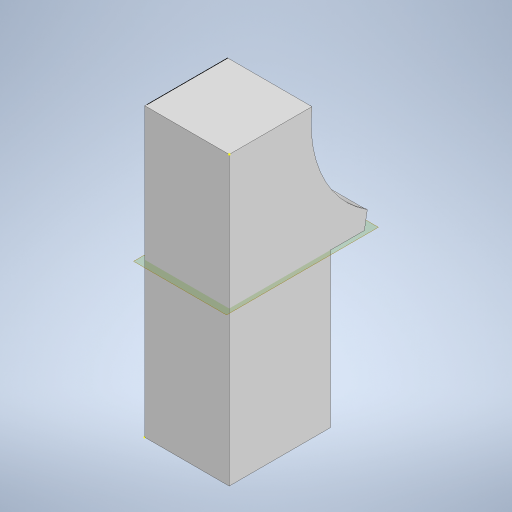
# Autodesk Inventor part: Pièce1
Saved by Autodesk Inventor 2023.1 (Build 271208000, 208)
## iProperties
Created: 2022-09-20
Part Number: Pièce1
Material: Générique
Document SubType Name: Sheet Metal
Designer: guiki
Density: 1 g/cm^3
Sheet Metal Rule: Par défaut_mm
Appearance: Par défaut
Author: guiki
Autodesk Inventor part; units mm, degrees
ref_plane "YZ Plane" through (0, 0, 0) normal (1, 0, 0) x (0, 1, 0)
ref_plane "XZ Plane" through (0, 0, 0) normal (0, 1, 0) x (-1, 0, 0)
ref_plane "XY Plane" through (0, 0, 0) normal (0, 0, 1) x (1, 0, 0)
sketch "Esquisse1" plane through (0, 0, 0) normal (0, 1, 0) x (-1, 0, 0)
  line L0 (0, 0) -> (500, 0)
  line L1 (500, 0) -> (500, -600)
  line L2 (500, -600) -> (0, -600)
  line L3 (0, -600) -> (0, 0)
  dimension "d0" = 500
  dimension "d1" = 600
  constraints: 8 end point, 2 parallel, 1 horizontal, 1 perpendicular
  measures "d0" distance of L1.end L2.end
  measures "d1" distance of L0.end L1.end
extrude "Extrusion1" add sketch "Esquisse1" along normal blind 1700
sketch "Esquisse3" plane through (0, 1700, 0) normal (0, 1, 0) x (1, 0, 0)
  line L0 (-500, 600) -> (-500, 0) projected
  line L1 (0, 600) -> (-500, 600) projected
  line L2 (-500, 13.2496) -> (0, 13.2496)
  line L3 (0, 13.2496) -> (0, 600)
  line L4 (0, 600) -> (-500, 600)
  line L5 (-500, 600) -> (-500, 13.2496)
  point P0 (0, 0)
  constraints: 8 end point, 2 parallel, 1 horizontal, 1 perpendicular, 1 point on line
extrude "Extrusion2" cut sketch "Esquisse3" against normal blind 790
sketch "Esquisse4" plane through (0, 910, 0) normal (0, 1, 0) x (1, 0, 0)
  line L0 (0, 13.2496) -> (-500, 13.2496) projected
  line L1 (0, 13.2496) -> (-10, 13.2496)
  line L2 (0, 600) -> (-500, 600) projected
  line L3 (-500, 600) -> (-490, 600)
  line L4 (-490, 600) -> (-490, 590)
  line L5 (-490, 590) -> (-10, 590)
  line L6 (-10, 590) -> (-10, 13.2496)
  line L7 (-10, 13.2496) -> (-490, 13.2496)
  line L8 (-490, 13.2496) -> (-490, 590)
  point P0 (0, 0)
  dimension "d7" = 10
  dimension "d8" = 10
  dimension "d9" = 10
  constraints: 14 end point, 2 parallel, 2 perpendicular, 2 point on line, 1 horizontal
  measures "d7" distance of L0.start L1.end
  measures "d8" distance of L2.end L3.end
  measures "d9" distance of L3.end L4.end
extrude "Extrusion3" cut sketch "Esquisse4" against normal blind 800
sketch "Esquisse5" plane through (0, 0, 0) normal (1, 0, 0) x (0, 0, -1)
  line L0 (600, 0) -> (600, 910) projected
  line L1 (600, 910) -> (800, 910)
  line L2 (800, 910) -> (817.3648, 1008.4808)
  line L3 (0, 0) -> (0, 1700) projected
  line L4 (0, 1700) -> (490, 1700)
  arc A0 (490, 1700) -> (817.3648, 1008.4808) centre (1204.9924, 1615.2302) ccw
  line L5 (13.2496, 1700) -> (13.2496, 910) projected
  line L6 (13.2496, 1700) -> (13.2496, 910)
  line L7 (13.2496, 910) -> (590, 910) projected
  line L8 (800, 910) -> (13.2496, 910)
  dimension "d12" = 200
  dimension "d13" = 100
  dimension "d14" = 100
  dimension "d15" = 490
  dimension "d16" = 720
  constraints: 10 end point, 3 horizontal, 2 point on circle, 1 centre point, 1 vertical
  measures "d12" distance of L0.end L1.end
  measures "d13" distance of L1.end L2.end
  measures "d14" angle of L2 L1
  measures "d15" distance of L3.end L4.end
  measures "d16" radius of A0
extrude "Extrusion4" add sketch "Esquisse5" against normal blind 10
sketch "Esquisse6" plane through (-500, 0, -600) normal (-1, 0, 0) x (0, 0, 1)
  line L0 (0, 0) -> (0, 910) projected
  line L1 (0, 910) -> (-200, 910) projected
  line L2 (0, 910) -> (-200, 910)
  line L3 (-200, 910) -> (-217.3648, 1008.4808)
  line L4 (586.7504, 910) -> (586.7504, 110) projected
  line L5 (0, 910) -> (586.7504, 910)
  line L6 (586.7504, 1700) -> (110, 1700) projected
  line L7 (586.7504, 910) -> (586.7504, 1700)
  line L8 (586.7504, 1700) -> (110, 1700)
  arc A0 (-217.3648, 1008.4808) -> (110, 1700) centre (-604.9924, 1615.2302) ccw
  point P0 (600, 0)
  dimension "d19" = 100
  dimension "d20" = 100
  constraints: 10 end point, 2 horizontal, 2 point on circle, 1 centre point, 1 collinear, 1 perpendicular
  measures "d19" distance of L1.end L3.end
  measures "d20" angle of L2 L3
sketch "Esquisse7" plane through (-500, 0, -600) normal (-1, 0, 0) x (0, 0, 1)
  line L0 (586.7504, 1700) -> (110, 1700) projected
  line L1 (110, 1700) -> (586.7504, 1700)
  line L2 (0, 0) -> (0, 910) projected
  line L3 (586.7504, 910) -> (10, 910) projected
  line L4 (0, 910) -> (586.7504, 910)
  line L5 (586.7504, 910) -> (586.7504, 1700)
  line L6 (0, 910) -> (-200, 910) projected
  line L7 (0, 910) -> (-200, 910)
  line L8 (-217.3648, 1008.4808) -> (-200, 910) projected
  line L9 (-200, 910) -> (-217.3648, 1008.4808)
  point P0 (600, 0)
  constraints: 10 end point, 2 collinear, 2 horizontal, 1 perpendicular
extrude "Extrusion5" add sketch "Esquisse6" against normal blind 10
ref_plane "Plan de construction1" through (0, 910, -800) normal (0, -1, 0) x (1, 0, 0)
sketch "Esquisse8" plane through (0, 910, -800) normal (0, -1, 0) x (1, 0, 0)
  line L0 (-10, 0) -> (-10, 200) projected
  line L1 (0, 200) -> (-500, 200) projected
  line L2 (-10, 0) -> (-490, 0)
  line L3 (-490, 0) -> (-490, 200)
  line L4 (-490, 200) -> (-10, 200)
  line L5 (-10, 200) -> (-10, 0)
  point P0 (0, 800)
  dimension "d23" = 480
  constraints: 8 end point, 2 parallel, 1 horizontal, 1 perpendicular, 1 point on line
  measures "d23" distance of L3.end L4.end
extrude "Extrusion6" add sketch "Esquisse8" against normal blind 10
sketch "Esquisse9" plane through (-490, 1008.4808, -817.3648) normal (0, -0.1736, -0.9848) x (-1, 0, 0)
  line L0 (-480, 541.3803) -> (-480, -1024.464) projected
  line L1 (0, -90.1519) -> (0, -100) projected
  line L2 (-480, -2.3513) -> (0, -2.3513)
  line L3 (0, -2.3513) -> (0, -90.1519)
  line L4 (0, -90.1519) -> (-480, -90.1519)
  line L5 (-480, -90.1519) -> (-480, -2.3513)
  point P0 (-490, -1135.0936)
  constraints: 8 end point, 2 parallel, 1 horizontal, 1 perpendicular, 1 point on line
extrude "Extrusion7" add sketch "Esquisse9" against normal blind 10
sketch "Esquisse10" plane through (0, 1700, 0) normal (0, 1, 0) x (1, 0, 0)
  point P0 (0, 0)
sketch "Esquisse11" plane through (0, 1700, 0) normal (0, 1, 0) x (1, 0, 0)
  line L0 (-500, 490) -> (-490, 490) projected
  line L1 (-490, 490) -> (-490, 10)
  line L2 (-490, 13.2496) -> (-490, 590) projected
  line L3 (-10, 590) -> (-10, 13.2496) projected
  line L4 (-10, 13.2496) -> (-490, 13.2496) projected
  line L5 (-10, 490) -> (-490, 490)
  line L6 (-490, 490) -> (-490, 13.2496)
  line L7 (-490, 13.2496) -> (-10, 13.2496)
  line L8 (-10, 13.2496) -> (-10, 490)
  point P0 (0, 0)
  dimension "d28" = 480
  constraints: 10 end point, 2 parallel, 1 collinear, 1 horizontal, 1 perpendicular, 1 point on line
  measures "d28" distance of L0.end L1.end
extrude "Extrusion8" add sketch "Esquisse11" against normal blind 10
sketch "Esquisse13" plane through (-490, 1006.1652, -816.9565) normal (0, 0.9848, -0.1736) x (1, 0, 0)
  line L0 (480, -10) -> (0, -10) projected
  line L1 (480, -10) -> (0, -10)
  line L2 (0, -10) -> (0, -210)
  line L3 (0, -210) -> (480, -210)
  line L4 (480, -210) -> (480, -10)
  point P0 (490, -629.8264)
  dimension "d33" = 480
  dimension "d34" = 200
  constraints: 8 end point, 2 parallel, 1 horizontal, 1 perpendicular
  measures "d33" distance of L3.end L2.end
  measures "d34" distance of L2.end L1.end
extrude "Extrusion9" add sketch "Esquisse13" against normal blind 10
equation "\"RayonPli\" = Epaisseur"
equation "\"LargeurGrugeage\" = Epaisseur"
equation "\"ProfondeurGrugeage\" = 0.5 * Epaisseur"
equation "\"TailleGrugeage\" = 4 * Epaisseur"
equation "\"RestesMinimum\" = 2 * Epaisseur"
equation "\"Rayondetransition\" = RayonPli"
equation "\"TailleRayonJacobi\" = RayonPli"
equation "\"TailleJeu\" = Epaisseur"
equation "\"Epaisseur\" = 0.5"
